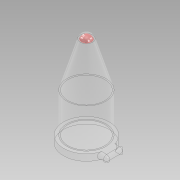
# Autodesk Inventor part: 6105_Example microcentrifuge tube_V1
Saved by Autodesk Inventor 2021 (Build 250183000, 183)
## iProperties
Created: 2023-05-09
Part Number: 6105_Example microcentrifuge tube_V1
Material: Polycarbonate, Clear
Document SubType Name: Modeling
Designer: Eli
Density: 1.2 g/cm^3
Appearance: Polycarbonate - Clear
Author: Eli
Autodesk Inventor part; units mm, degrees
ref_plane "YZ Plane" through (0, 0, 0) normal (1, 0, 0) x (0, 1, 0)
ref_plane "XZ Plane" through (0, 0, 0) normal (0, 1, 0) x (-1, 0, 0)
ref_plane "XY Plane" through (0, 0, 0) normal (0, 0, 1) x (1, 0, 0)
sketch "Sketch1" plane through (0, 0, 0) normal (0, 0, 1) x (1, 0, 0)
  line L0 (0, 10) -> (3, 0)
  line L1 (3, 0) -> (3, -6)
  line L2 (3, -6) -> (0, -6)
  line L3 (0, -6) -> (0, 10)
  arc A0 (0.9578, 6.8072) -> (0, 7.5199) centre (0, 6.5199) ccw
  point P0 (0, 0)
  dimension "d0" = 3
  dimension "d1" = 6
  dimension "d2" = 10
  dimension "d4" = 1
  constraints: 8 end point, 4 point on line, 2 perpendicular, 2 point on circle, 1 centre point, 1 horizontal alignment, 1 line through centre, 1 tangent, 1 vertical
  measures "d0" distance between parallel lines of L3 L1
  measures "d1" distance of L0.end L1.end
  measures "d2" vertical distance of L0.start L0.end
  measures "d4" radius of A0
revolve "Revolution1" add sketch "Sketch1" angle 360 about axis through (0, -6, 0) along (0, 1, 0) contours L0 L1 L2 L3 A0
shell "Shell1" thickness 0.2 removed faces 1 at (-1.1424, -6, -0.935)
sketch "Sketch2" plane through (0, 0, 0) normal (1, 0, 0) x (0, 1, 0)
  line L0 (-0.0294, 2.8) -> (-0.0294, -2.8) projected
  line L1 (-6, -2.8) -> (-6, 2.8) projected
  line L2 (6.7498, 0.7663) -> (6.7498, -0.7663) projected
  line L3 (-0.0294, 2.8) -> (-0.0294, -2.8) projected
  line L4 (6.7498, 0.7663) -> (6.7498, -0.7663) projected
  arc A0 (6.7498, -0.7663) -> (6.7498, 0.7663) centre (6.5199, 0) ccw projected
  line L5 (7.3199, 0) -> (6.7498, 0)
  point P0 (0, 0)
  constraints: 2 end point, 1 midpoint, 1 point on circle
revolve "Revolution2" add sketch "Sketch2" angle 360 about axis through (0, 7.3199, 0) along (0, -1, 0) separate body picked at (6.8021, 0.4889) contours A0 L5 L2
sketch "Sketch3" plane through (0, -6, 0) normal (0, -1, 0) x (1, 0, 0)
  circle A0 centre (0, 0) radius 3 projected
  circle A1 centre (0, 0) radius 3 projected
  line L0 (2.5981, 1.5) -> (4.5981, 1.5)
  line L1 (4.5981, 1.5) -> (4.5981, -1.5)
  line L2 (4.5981, -1.5) -> (2.5981, -1.5)
  line L3 (2.5981, -1.5) -> (2.5981, 1.5)
  circle A2 centre (0, 0) radius 3.5
  point P0 (0, 0)
  point P1 (4.5981, 0)
  point P2 (3.1623, 1.5)
  point P3 (3.1623, -1.5)
  dimension "d7" = 3
  dimension "d8" = 2
  dimension "d11" = 0.5
  constraints: 8 end point, 2 parallel, 1 centre point, 1 horizontal, 1 horizontal alignment, 1 midpoint, 1 perpendicular, 2 other
  measures "d7" distance between parallel lines of L2 L0
  measures "d8" distance of L0.start L0.end
  measures "d11" radial gap between concentric circles of A0 A2
extrude "Extrusion1" add sketch "Sketch3" along normal blind 1 bodies 1
fillet "Fillet1" radius 0.5 2 edges at (4.5981, -6.5, 1.5) (4.5981, -6.5, -1.5)
fillet "Fillet2" radius 0.5 10 edges at (4.4516, -6, 1.3536) (3.6302, -6, 1.5) (4.4516, -6, -1.3536) (3.6302, -6, -1.5) (4.5981, -6, 0) (4.4516, -7, 1.3536) (3.6302, -7, 1.5) (4.4516, -7, -1.3536) (3.6302, -7, -1.5) (4.5981, -7, 0)
body "Solid1"
body "Solid2"
